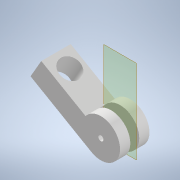
# Autodesk Inventor part: Palanca servo_dedo_1
Saved by Autodesk Inventor 2020 (Build 240168000, 168)
## iProperties
Created: 2021-08-16
Part Number: Palanca servo_dedo_1
Material: Generic
Document SubType Name: Modeling
Designer: chalo
Density: 1 g/cm^3
Appearance: Default
Author: chalo
Autodesk Inventor part; units mm, degrees
ref_plane "YZ Plane" through (0, 0, 0) normal (1, 0, 0) x (0, 1, 0)
ref_plane "XZ Plane" through (0, 0, 0) normal (0, 1, 0) x (-1, 0, 0)
ref_plane "XY Plane" through (0, 0, 0) normal (0, 0, 1) x (1, 0, 0)
sketch "Sketch1" plane through (0, 0, 0) normal (0, 0, 1) x (1, 0, 0)
  circle A0 centre (0, -7.23) radius 0.5 projected
  circle A1 centre (0, -7.23) radius 3.75
  point P0 (0, 0)
  dimension "d0" = 7.5
  constraints: 1 centre point, 1 coincident
  measures "d0" diameter of A1
extrude "Extrusion1" add sketch "Sketch1" along normal blind 2
ref_plane "Work Plane1" through (0, 0, -1.75) normal (0, 0, -1) x (-1, 0, 0)
sketch "Sketch2" plane through (0, 0, -1.75) normal (0, 0, -1) x (-1, 0, 0)
  circle A0 centre (0, -7.23) radius 0.5 projected
  circle A1 centre (0, -7.23) radius 3.75 projected
  circle A2 centre (0, -7.23) radius 0.5 projected
  point P0 (0, 0)
extrude "Extrusion2" add sketch "Sketch2" along normal blind 2
sketch "Sketch3" plane through (0, -7.23, 2) normal (0, 0, 1) x (1, 0, 0)
  line L0 (-1.7434, -1.6216) -> (-2.9, 11.6822) construction
  arc A0 (-1.7434, -1.6216) -> (1.7434, -1.6216) centre (0, -1.47) ccw construction
  line L1 (1.7434, -1.6216) -> (2.9, 11.6822) construction
  arc A1 (2.9, 11.6822) -> (-2.9, 11.6822) centre (0, 13.98) ccw construction
  circle A2 centre (0, 13.98) radius 2.7 construction
  circle A3 centre (0, 6.21) radius 0.5 construction
  circle A4 centre (0, 8.28) radius 0.5 construction
  circle A5 centre (0, -2.07) radius 0.5 construction
  circle A6 centre (0, 0) radius 0.5 construction
  circle A7 centre (0, 2.07) radius 0.5 construction
  circle A8 centre (0, 4.14) radius 0.5 construction
  circle A9 centre (0, 0) radius 3.75 projected
  circle A10 centre (0, 0) radius 3.75 projected
  line L2 (-2.9991, 2.2512) -> (-11.6594, 7.2512)
  line L3 (-1.875, -3.2476) -> (-13.7594, 3.6139)
  line L4 (-12.9585, 11.9353) -> (6.9601, 0.4353) projected
  line L5 (-11.6594, 7.2512) -> (-13.7594, 3.6139)
  point P0 (0, 7.23)
  point P1 (-1.875, -3.2476)
  dimension "d5" = 90
  dimension "d6" = 4.2
  dimension "d7" = 10
  constraints: 6 end point, 2 parallel, 2 point on circle, 1 tangent
  measures "d5" angle of L5 L2
  measures "d6" distance of L2.end L3.end
  measures "d7" distance of L2.start L2.end
extrude "Extrusion3" add sketch "Sketch3" against normal up to surface (5.75 mm away) contours A9 L3 L5 L2
sketch "Sketch4" plane through (-11.6594, 0.0212, 2) normal (0.5, 0.8660254, 0) x (0.8660254, -0.5, 0)
  line L0 (10, 5.75) -> (0, 5.75) projected
  line L1 (0, 0) -> (0, 5.75) projected
  line L2 (10, 0) -> (0, 0) projected
  line L3 (10, 2) -> (10, 0) projected
  line L4 (10, 2) -> (10, 3.75) projected
  line L5 (10, 5.75) -> (10, 3.75) projected
  circle A0 centre (2.5, 3) radius 1.6
  point P0 (10.1079, 2)
  dimension "d10" = 3.2
  dimension "d11" = 2.5
  dimension "d12" = 3
  constraints: 1 centre point
  measures "d10" diameter of A0
  measures "d11" distance from line of L1 A0.centre
  measures "d12" distance from line of L2 A0.centre
extrude "Extrusion4" cut sketch "Sketch4" against normal through all contours A0
body "Solid1"
